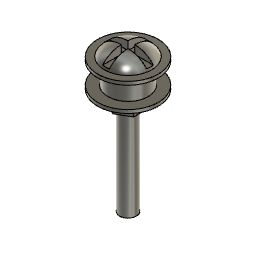
b70abd27-0663-4f6c-be06-7210419bfb21 (Autodesk Fusion 360 design; units mm, degrees)
Autodesk Fusion 360 part; units mm, degrees
sketch "Sketch1" plane through (0, 0, 0) normal (0, 0, 1) x (1, 0, 0)
  circle A0 centre (0, 0) radius 6
  dimension "d1" = 12
  constraint coincident A0.centre origin
  measures "d1" diameter of A0
extrude "Extrude1" add sketch "Sketch1" along normal blind 6.3 makes body 1
sketch "Sketch2" plane through (0, 0, 6.3) normal (0, 0, 1) x (-1, 0, 0)
  circle A0 centre (0, 0) radius 6
  circle A1 centre (0, 0) radius 9
  dimension "d4" = 18
  constraint concentric A0 A1
  measures "d4" diameter of A1
extrude "Extrude2" add sketch "Sketch2" along normal blind 1 contours A0 | A1 bodies 1
sketch "Sketch3" plane through (0, 0, 0) normal (0, 0, -1) x (1, 0, 0)
  circle A0 centre (0, 0) radius 6
  circle A1 centre (0, 0) radius 9
  dimension "d7" = 18
  constraint concentric A0 A1
  measures "d7" diameter of A1
extrude "Extrude3" add sketch "Sketch3" along normal blind 1 contours A0 | A1 bodies 1
sketch "Sketch4" plane through (0, 0, -1) normal (0, 0, -1) x (1, 0, 0)
  circle A0 centre (0, 0) radius 9
  circle A1 centre (0, 0) radius 2.5
  dimension "d10" = 5
  constraint coincident A0.centre A1.centre
  measures "d10" diameter of A1
extrude "Extrude4" cut sketch "Sketch4" against normal blind 16 contours A1 bodies 1
ref_plane "WorkPlane1" through (0, 0, 7.4) normal (0, 0, 1) x (-1, 0, 0)
sketch "Sketch5" plane through (0, 0, 7.4) normal (0, 0, 1) x (1, 0, 0)
  circle A0 centre (0, 0) radius 7
  dimension "d14" = 14
  constraint coincident A0.centre origin
  measures "d14" diameter of A0
extrude "Extrude5" add sketch "Sketch5" along normal blind 3 separate body makes body 2
fillet "Fillet1" radius 7 1 edges at (-6.5263, -2.5313, 10.4) on bodies 2
sketch "Sketch6" plane through (0, 0, 10.4) normal (0, 0, 1) x (-1, 0, 0)
  circle A0 centre (0, 0) radius 1.2554
  line L0 (-14, 1) -> (16, 1)
  line L1 (16, 1) -> (16, -1)
  line L2 (16, -1) -> (-14, -1)
  line L3 (-14, -1) -> (-14, 1)
  line L4 (-1, 13.5164) -> (1, 13.5164)
  line L5 (1, 13.5164) -> (1, -12)
  line L6 (1, -12) -> (-1, -12)
  line L7 (-1, -12) -> (-1, 13.5164)
  dimension "d18" = 2
  dimension "d19" = 2
  dimension "d20" = 1
  dimension "d21" = 1
  constraint horizontal L0
  constraint vertical L1
  constraint horizontal L2
  constraint vertical L3
  constraint horizontal L4
  constraint vertical L5
  constraint horizontal L6
  constraint vertical L7
  measures "d18" distance of L0.end L1.end
  measures "d19" distance of L5.end L6.end
  measures "d20" horizontal distance of A0.centre L4.start
  measures "d21" vertical distance of A0.centre L0.end
extrude "Extrude6" cut sketch "Sketch6" against normal blind 2.5 bodies 2
sketch "Sketch7" plane through (0, 0, -1) normal (0, 0, -1) x (1, 0, 0)
  circle A0 centre (0, 0) radius 2.5
  circle A1 centre (0, 0) radius 9
  circle A2 centre (0, 0) radius 2.55
  dimension "d24" = 5.1
  constraint coincident A0.centre A1.centre
  measures "d24" diameter of A2
extrude "Extrude7" cut sketch "Sketch7" against normal blind 8.3 contours A2 bodies 1
sketch "Sketch8" plane through (0, 0, 7.4) normal (0, 0, -1) x (1, 0, 0)
  circle A0 centre (0, 0) radius 7
  circle A1 centre (0, 0) radius 2.5
  dimension "d27" = 5
  constraint concentric A0 A1
  measures "d27" diameter of A1
extrude "Extrude8" add sketch "Sketch8" along normal blind 40 contours A1 bodies 2
ref_plane "WorkPlane2" through (0, 0, -1.1) normal (0, 0, -1) x (1, 0, 0)
sketch "Sketch9" plane through (0, 0, -1.1) normal (0, 0, -1) x (1, 0, 0)
  circle A0 centre (0, 0) radius 2.5
  circle A1 centre (0, 0) radius 2.5
  line L0 (4, 2.3094) -> (0, 4.6188)
  line L1 (0, 4.6188) -> (-4, 2.3094)
  line L2 (-4, 2.3094) -> (-4, -2.3094)
  line L3 (-4, -2.3094) -> (0, -4.6188)
  line L4 (0, -4.6188) -> (4, -2.3094)
  line L5 (4, -2.3094) -> (4, 2.3094)
  circle A2 centre (0, 0) radius 2.6
  dimension "d31" = 4
  dimension "d32" = 5.2
  constraint coincident A0.centre A1.centre
  measures "d31" distance of A0.centre L5
  measures "d32" diameter of A2
extrude "Extrude9" add sketch "Sketch9" along normal blind 4 separate body contours L0 L1 L2 L3 L4 L5 makes body 3
